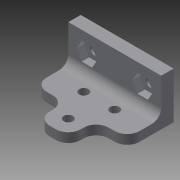
# Autodesk Inventor part: ChimeraMountingBlock
Saved by Autodesk Inventor 2015 (Build 190159000, 159)
## iProperties
Created: 2014-11-30
Part Number: ChimeraMountingBlock
Material: Generic
Document SubType Name: Modeling
Designer: Jack
Density: 1 g/cm^3
Appearance: Default
Author: Jack
Autodesk Inventor part; units mm, degrees
ref_plane "YZ Plane" through (0, 0, 0) normal (1, 0, 0) x (0, 1, 0)
ref_plane "XZ Plane" through (0, 0, 0) normal (0, 1, 0) x (-1, 0, 0)
ref_plane "XY Plane" through (0, 0, 0) normal (0, 0, 1) x (1, 0, 0)
sketch "Sketch1" plane through (0, 0, 0) normal (0, 0, 1) x (1, 0, 0)
  circle A0 centre (0, 0) radius 1.5
  circle A1 centre (10, 0) radius 1.5
  circle A2 centre (5, -10) radius 1.5
  line L0 (-10, 9) -> (20, 9)
  circle A3 centre (-4, -8) radius 1.5 construction
  circle A4 centre (-4, -18) radius 1.5 construction
  circle A5 centre (14, -8) radius 1.5 construction
  circle A6 centre (14, -18) radius 1.5 construction
  line L1 (-10, 9) -> (-10, -6)
  line L2 (-10, -6) -> (0, -6)
  line L3 (0, -6) -> (0, -15)
  line L4 (0, -15) -> (10, -15)
  line L5 (10, -15) -> (10, -6)
  line L6 (10, -6) -> (20, -6)
  line L7 (20, -6) -> (20, 9)
  dimension "d0" = 3
  dimension "d1" = 5
  dimension "d2" = 10
  dimension "d3" = 10
  dimension "d4" = 30
  dimension "d5" = 9
  dimension "d6" = 10
  dimension "d7" = 10
  dimension "d8" = 18
  dimension "d9" = 6
  dimension "d10" = 3
  dimension "d11" = 17
  dimension "d16" = 15
  dimension "d17" = 10
  dimension "d18" = 5
  dimension "d19" = 5
  constraints: 16 end point, 7 centre point, 5 equal radius, 5 perpendicular, 3 horizontal alignment, 2 point on line, 2 vertical alignment, 1 coincident, 1 horizontal, 1 vertical
  measures "d0" diameter of A0
  measures "d1" horizontal distance of point (0, 0) A2.centre
  measures "d2" distance of point (0, 0) A1.centre
  measures "d3" vertical distance of A1.centre A2.centre
  measures "d4" distance of L0.start L0.end
  measures "d5" distance from line of L0 point (0, 0)
  measures "d6" horizontal distance of point (0, 0) L0.start
  measures "d7" distance of A3.centre A4.centre
  measures "d8" distance of A6.centre A4.centre
  measures "d9" horizontal distance of L0.start A3.centre
  measures "d10" diameter of A3
  measures "d11" distance from line of L0 A5.centre
  measures "d16" distance between parallel lines of L0 L2
  measures "d17" distance between parallel lines of L5 L3
  measures "d18" distance from line of A2.centre L5
  measures "d19" distance from line of L4 A2.centre
extrude "Extrusion1" add sketch "Sketch1" along normal blind 3
fillet "Fillet2" radius 4 6 edges at (0, -6, 1.5) (10, -6, 1.5) (10, -15, 1.5) (0, -15, 1.5) (-10, -6, 1.5) (20, -6, 1.5)
sketch "Sketch2" plane through (0, 0, 3) normal (0, 0, 1) x (1, 0, 0)
  line L0 (20, -2) -> (20, 9) projected
  line L1 (20, 9) -> (-10, 9) projected
  line L2 (-10, 9) -> (-10, -2) projected
  line L3 (-10, 5) -> (20, 5)
  dimension "d21" = 4
  constraints: 2 end point, 2 point on line, 1 perpendicular
  measures "d21" distance between parallel lines of L1 L3
extrude "Extrusion2" add sketch "Sketch2" along normal blind 12
sketch "Sketch3" plane through (-10, 5, 3) normal (0, -1, 0) x (1, 0, 0)
  line L0 (0, 0) -> (0, 12) projected
  circle A0 centre (6, 6) radius 1.5
  circle A1 centre (24, 6) radius 1.5
  line L1 (0, -3) -> (30, -3) projected
  point P0 (10, -3)
  dimension "d24" = 18
  dimension "d25" = 6
  dimension "d26" = 9
  dimension "d27" = 3
  constraints: 2 centre point, 1 equal radius, 1 horizontal alignment
  measures "d24" distance of A1.centre A0.centre
  measures "d25" distance from line of L0 A0.centre
  measures "d26" distance from line of L1 A0.centre
  measures "d27" diameter of A0
extrude "Extrusion3" cut sketch "Sketch3" against normal up to next
sketch "Sketch4" plane through (-10, 5, 3) normal (0, -1, 0) x (1, 0, 0)
  circle A0 centre (6, 6) radius 1.5 projected
  circle A1 centre (24, 6) radius 1.5 projected
  line L0 (9.3486, 6) -> (7.6743, 3.1)
  line L1 (7.6743, 3.1) -> (4.3257, 3.1)
  line L2 (4.3257, 3.1) -> (2.6514, 6)
  line L3 (2.6514, 6) -> (4.3257, 8.9)
  line L4 (4.3257, 8.9) -> (7.6743, 8.9)
  line L5 (7.6743, 8.9) -> (9.3486, 6)
  circle A2 centre (24, 6) radius 1.5 projected
  line L6 (27.3486, 6) -> (25.6743, 3.1)
  line L7 (25.6743, 3.1) -> (22.3257, 3.1)
  line L8 (22.3257, 3.1) -> (20.6514, 6)
  line L9 (20.6514, 6) -> (22.3257, 8.9)
  line L10 (22.3257, 8.9) -> (25.6743, 8.9)
  line L11 (25.6743, 8.9) -> (27.3486, 6)
  point P0 (10, -3)
  dimension "d30" = 5.8
  constraints: 24 end point, 2 coincident, 2 horizontal, 1 collinear, 26 other
  measures "d30" distance between parallel lines of L1 L4
extrude "Extrusion4" cut sketch "Sketch4" against normal blind 2.4
fillet "Fillet3" radius 3 1 edges at (5, 5, 3)
body "Solid1"
